Picture Frame Holder (Autodesk Fusion 360 design; units mm, degrees)
Autodesk Fusion 360 part; units mm, degrees
sketch "Sketch1" plane through (0, 0, 0) normal (0, 0, 1) x (1, 0, 0)
  line L0 (0, 0) -> (20, 0)
  line L1 (20, 0) -> (20, 30)
  line L2 (20, 30) -> (0, 30)
  line L3 (0, 30) -> (0, 0)
  line L4 (0, 0) -> (20, 0)
  line L5 (20, 0) -> (20, 10)
  line L6 (20, 10) -> (0, 10)
  line L7 (0, 10) -> (0, 0)
  circle A0 centre (6, 5) radius 0.75
  circle A1 centre (14, 5) radius 0.75
  dimension "d1" = 20
  dimension "d2" = 30
  dimension "d3" = 10
  dimension "d4" = 1.5
  dimension "d5" = 5
  dimension "d6" = 6
  dimension "d7" = 1.5
  dimension "d8" = 5
  dimension "d9" = 6
  constraint horizontal L0
  constraint vertical L1
  constraint horizontal L2
  constraint vertical L3
  constraint coincident L0.start L3.end
  constraint horizontal L4
  constraint vertical L5
  constraint horizontal L6
  constraint vertical L7
  measures "d1" distance of L0.start L0.end
  measures "d2" distance of L0.start L2.end
  measures "d3" distance of L0.start L6.end
  measures "d4" diameter of A0
  measures "d5" distance of L6 A0.centre
  measures "d6" distance of L7 A0.centre
  measures "d7" diameter of A1
  measures "d8" distance of L6 A1.centre
  measures "d9" distance of L5 A1.centre
extrude "Extrude1" add sketch "Sketch1" along normal blind 1
